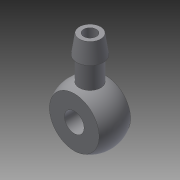
# Autodesk Inventor part: Fuelintake
Saved by Autodesk Inventor 2015 (Build 190159000, 159)
## iProperties
Created: 2016-02-20
Part Number: Fuelintake
Material: Generic
Document SubType Name: Modeling
Designer: Owner
Density: 1 g/cm^3
Appearance: Default
Author: Owner
Autodesk Inventor part; units mm, degrees
ref_plane "YZ Plane" through (0, 0, 0) normal (1, 0, 0) x (0, 1, 0)
ref_plane "XZ Plane" through (0, 0, 0) normal (0, 1, 0) x (-1, 0, 0)
ref_plane "XY Plane" through (0, 0, 0) normal (0, 0, 1) x (1, 0, 0)
sketch "Sketch1" plane through (0, 0, 0) normal (0, 1, 0) x (-1, 0, 0)
  circle A0 centre (0, 0) radius 4.7498
  line L0 (4.7498, 0) -> (-4.7498, 0)
  dimension "d0" = 9.4996
  constraints: 2 end point, 2 point on circle, 1 centre point, 1 coincident, 1 horizontal
  measures "d0" diameter of A0
revolve "Revolution1" add sketch "Sketch1" angle 360 about axis through (-4.7498, 0, 0) along (1, 0, 0) picked at (1.1851, -1.0499) contours A0 L0
sketch "Sketch2" plane through (0, 0, 0) normal (1, 0, 0) x (0, 1, 0)
  circle A0 centre (0, 0) radius 4.7498 projected
  line L0 (-4.0136, -2.54) -> (4.0136, -2.54)
  line L1 (-4.0136, 2.54) -> (4.0136, 2.54)
  constraints: 4 end point, 4 point on circle, 2 horizontal
extrude "Extrusion1" cut sketch "Sketch2" along normal mid plane 25.4 contours L1 A0 | A0 L0
hole "Hole1" at (0, 0, -2.54) direction (0, 0, 1) diameter 3.175 end through all
sketch "Sketch3" plane through (0, 0, 0) normal (1, 0, 0) x (0, 1, 0)
  line L0 (4.0136, -2.54) -> (-4.0136, -2.54) projected
  line L1 (-4.0136, 2.54) -> (4.0136, 2.54) projected
  line L2 (0, 0) -> (4.4196, 0) construction
  line L3 (4.4196, 0) -> (4.4196, -1.74)
  arc A0 (4.0136, -2.54) -> (-4.0136, -2.54) centre (0, 0) ccw projected
  line L4 (4.4196, 0) -> (11.2522, 0)
  line L5 (11.2522, 0) -> (11.2522, -1.7272)
  line L6 (4.4196, -1.74) -> (8.2042, -1.74)
  line L7 (8.2042, -1.74) -> (8.2042, -2.1718)
  line L8 (8.2042, -2.1718) -> (11.2522, -1.7272)
  dimension "d6" = 4.4196
  dimension "d7" = 6.8326
  dimension "d8" = 1.7272
  dimension "d9" = 3.7846
  dimension "d10" = 0.4318
  constraints: 14 end point, 3 horizontal, 2 vertical, 1 perpendicular, 1 point on circle
  measures "d6" distance of L2.start L2.end
  measures "d7" distance of L2.end L4.end
  measures "d8" distance of L4.end L5.end
  measures "d9" distance of L3.end L6.end
  measures "d10" distance of L6.end L7.end
revolve "Revolution2" add sketch "Sketch3" angle 360 about axis through (0, 4.4196, 0) along (0, 1, 0) contours L3 L4 A0 | A0 L4 L5 L8 L7 L6
hole "Hole2" at (0, 11.2522, 0) direction (0, -1, 0) diameter 2.0574 end up to face face through (0, 0, 11.8228) facing (0, 0, -1) round with radius 1.5875 far side yes clearance for "Flat Head Machine Screw (82)" size "#1" standard "Ansi Unified Screw Threads"
body "Solid1"
